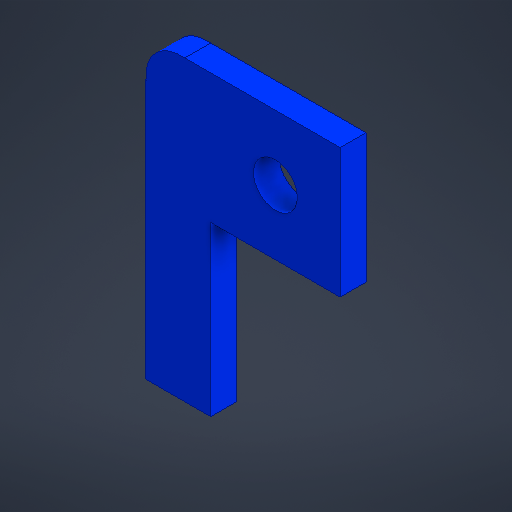
# Autodesk Inventor part: Belt Holders
Saved by Autodesk Inventor 2025.1 (Build 291241000, 241)
## iProperties
Created: 2024-10-17
Part Number: Belt Holders
Material: Generic
Document SubType Name: Modeling
Designer: jerem
Density: 1 g/cm^3
Appearance: Default
Author: jerem
## iProperties of the stored document Belt Holders_3DPrint.ipt
Created: 2024-11-18
Part Number: Belt Holders_3DPrint
Material: Generic
Document SubType Name: Modeling
Designer: jerem
Density: 1 g/cm^3
Appearance: Default
Author: jerem
Autodesk Inventor part; units mm, degrees
ref_plane "YZ Plane" through (0, 0, 0) normal (1, 0, 0) x (0, 1, 0)
ref_plane "XZ Plane" through (0, 0, 0) normal (0, 1, 0) x (-1, 0, 0)
ref_plane "XY Plane" through (0, 0, 0) normal (0, 0, 1) x (1, 0, 0)
sketch "Sketch1" plane through (0, 0, 0) normal (0, 0, 1) x (1, 0, 0)
  line L0 (0, 0) -> (0, 23)
  line L1 (0, 23) -> (15, 23)
  line L2 (15, 23) -> (15, 13)
  line L3 (15, 13) -> (5, 13)
  line L4 (5, 13) -> (5, 0)
  line L5 (5, 0) -> (0, 0)
  circle A0 centre (10, 18) radius 1.7
  point P0 (15, 18)
  dimension "d14" = 23
  dimension "d15" = 15
  dimension "d16" = 10
  dimension "d17" = 10
  dimension "d18" = 3.4
  dimension "d19" = 5
  dimension "d20" = 5
  constraints: 12 end point, 5 perpendicular, 1 centre point, 1 midpoint, 1 vertical
  measures "d14" distance of L0.start L0.end
  measures "d15" distance of L0.end L1.end
  measures "d16" distance of L1.end L2.end
  measures "d17" distance of L2.end L3.end
  measures "d18" diameter of A0
  measures "d19" distance of point (15, 18) A0.centre
  measures "d20" distance from line of L1 A0.centre
extrude "Extrusion1" add sketch "Sketch1" along normal blind 2
fillet "Fillet1" radius 3 1 edges at (0, 23, 1) curvature continuous yes
body "Solid1"
